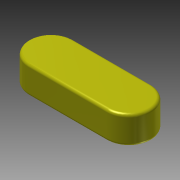
# Autodesk Inventor part: 装填盘轴键
Saved by Autodesk Inventor 2015 (Build 190159000, 159)
## iProperties
Created: 2017-05-04
Part Number: 装填盘轴键
Material: 常规
Document SubType Name: Modeling
Designer: Administrator
Density: 1 g/cm^3
Appearance: 黄色
Author: Administrator
Autodesk Inventor part; units mm, degrees
ref_plane "YZ Plane" through (0, 0, 0) normal (1, 0, 0) x (0, 1, 0)
ref_plane "XZ Plane" through (0, 0, 0) normal (0, 1, 0) x (-1, 0, 0)
ref_plane "XY Plane" through (0, 0, 0) normal (0, 0, 1) x (1, 0, 0)
sketch "草图1" plane through (0, 0, 0) normal (0, 0, 1) x (1, 0, 0)
  line L0 (0, 0) -> (14, 0)
  line L1 (14, 0) -> (14, -8)
  line L2 (14, -8) -> (0, -8)
  line L3 (0, -8) -> (0, 0)
  arc A0 (14, -8) -> (14, 0) centre (14, -4) ccw
  arc A1 (0, 0) -> (0, -8) centre (0, -4) ccw
  dimension "d0" = 14
  dimension "d1" = 8
  constraints: 8 end point, 4 point on circle, 4 tangent, 2 centre point, 2 parallel, 1 coincident, 1 horizontal, 1 perpendicular
  measures "d0" distance of L0.start L0.end
  measures "d1" distance of L0.end L1.end
extrude "拉伸1" add sketch "草图1" against normal blind 5
fillet "圆角1" radius 0.5 8 edges at (7, 0, 0) (-4, -4, 0) (7, -8, 0) (18, -4, 0) (7, -8, -5) (-4, -4, -5) (7, 0, -5) (18, -4, -5)
